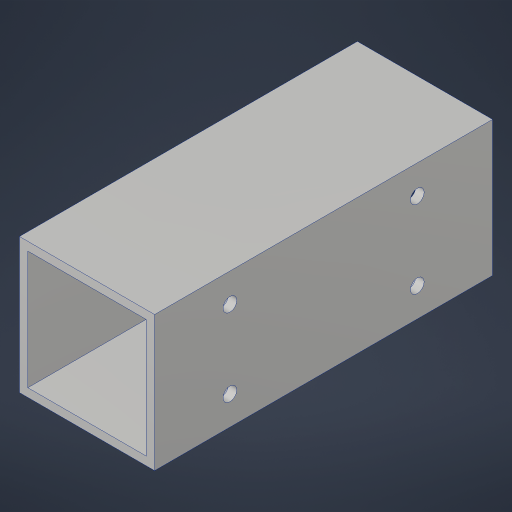
# Autodesk Inventor part: EL2-A-007
Saved by Autodesk Inventor 2023.4 (Build 274418000, 418)
## iProperties
RuleStatus: InUse
Created: 2025-01-19
Part Number: EL2-A-007
Material: Aluminum 6061
Document SubType Name: Modeling
Designer: brand
Mass: 103.699 g
Surface Area: 254.032 cm^2
Volume: 38.4072 cm^3
Density: 2.7 g/cm^3
Appearance: Aluminum - Flat
AfterDocNew0: SHOW
AfterDocOpen0: SHOW
Author: brand
Autodesk Inventor part; units mm, degrees
ref_plane "YZ Plane" through (0, 0, 0) normal (1, 0, 0) x (0, 1, 0)
ref_plane "XZ Plane" through (0, 0, 0) normal (0, 1, 0) x (-1, 0, 0)
ref_plane "XY Plane" through (0, 0, 0) normal (0, 0, 1) x (1, 0, 0)
sketch "Sketch1" plane through (0, 0, 0) normal (0, 0, 1) x (1, 0, 0)
  line L0 (-25.4, -25.4) -> (25.4, -25.4)
  line L1 (25.4, -25.4) -> (25.4, 25.4)
  line L2 (25.4, 25.4) -> (-25.4, 25.4)
  line L3 (-25.4, 25.4) -> (-25.4, -25.4)
  line L4 (-25.4, -25.4) -> (25.4, 25.4) construction
  line L5 (25.4, -25.4) -> (-25.4, 25.4) construction
  line L6 (-22.225, 22.225) -> (22.225, 22.225)
  line L7 (22.225, 22.225) -> (22.225, -22.225)
  line L8 (22.225, -22.225) -> (-22.225, -22.225)
  line L9 (-22.225, -22.225) -> (-22.225, 22.225)
  point P0 (0, 0)
  dimension "width" = 50.8
  dimension "height" = 50.8
  dimension "thickness" = 3.175
  constraints: 20 end point, 4 parallel, 2 midpoint, 2 perpendicular, 1 horizontal, 3 other
  measures "width" distance of L2.end L1.end
  measures "height" distance of L1.end L0.end
  measures "thickness" distance between parallel lines of L2 L6
extrude "Extrusion1" add sketch "Sketch1" along normal mid plane 127
sketch "Sketch2" plane through (25.4, -25.4, 63.5) normal (1, 0, 0) x (0, 0, -1)
  line L0 (127, 50.8) -> (127, 0) construction
  line L1 (127, 0) -> (0, 0) construction
  line L2 (0, 0) -> (0, 50.8) construction
  line L3 (0, 50.8) -> (127, 50.8) construction
  circle A0 centre (63.5, 25.4) radius 38.1 construction
  line L4 (48.9198, 60.5998) -> (78.0802, 60.5998) construction
  point P0 (78.0802, 60.5998)
  point P1 (28.3002, 39.9802)
  point P2 (28.3002, 10.8198)
  point P3 (48.9198, -9.7998)
  point P4 (78.0802, -9.7998)
  point P5 (98.6998, 10.8198)
  point P6 (98.6998, 39.9802)
  dimension "d5" = 76.2
  dimension "d8" = 360
  constraints: 2 coincident, 2 end point, 2 point on circle, 1 centre point, 1 horizontal, 9 other
  measures "d5" diameter of A0
hole "Hole1" at (25.4, 35.1998, -14.5802) at (25.4, 35.1998, 14.5802) at (25.4, 14.5802, 35.1998) at (25.4, -14.5802, 35.1998) at (25.4, -35.1998, 14.5802) at (25.4, -35.1998, -14.5802) at (25.4, -14.5802, -35.1998) at (25.4, 14.5802, -35.1998) direction (-1, 0, 0) diameter 5.1054 depth 3.175 tip angle 118 clearance for "Flat Head Machine Screw (82)" size "#10" standard "Ansi Unified Screw Threads"
body "Solid1"
